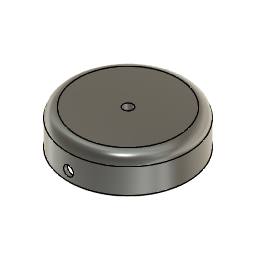
cap tesla coil (Autodesk Fusion 360 design; units mm, degrees)
Autodesk Fusion 360 part; units mm, degrees
sketch "Sketch1" plane through (0, 0, 0) normal (0, 0, 1) x (1, 0, 0)
  circle A0 centre (0, 0) radius 23
  circle A1 centre (0, 0) radius 24.5
  dimension "d1" = 46
  dimension "d2" = 49
  constraint coincident A0.centre A1.centre
  measures "d1" diameter of A0
  measures "d2" diameter of A1
extrude "Extrude1" add sketch "Sketch1" along normal blind 12
sketch "Sketch2" plane through (0, 0, 12) normal (0, 0, 1) x (-1, 0, 0)
  circle A0 centre (0, 0) radius 23
  circle A1 centre (0, 0) radius 24.5
  circle A2 centre (0, 0) radius 2
  circle A3 centre (0, 0) radius 24.5
  dimension "d5" = 4
  constraint coincident A0.centre A1.centre
  measures "d5" diameter of A2
extrude "Extrude2" add sketch "Sketch2" along normal blind 3 contours A0 | A1 A3
fillet "Fillet1" radius 4 1 edges at (22.842, 8.8596, 15)
sketch "Sketch3" plane through (0, 0, 0) normal (0, 1, 0) x (1, 0, 0)
  line L0 (0, 0) -> (0, -4.5)
  circle A0 centre (0, -4.5) radius 2
  dimension "d10" = 4.5
  dimension "d11" = 4
  constraint coincident L0.start origin
  constraint vertical L0
  constraint coincident L0.end A0.centre
  measures "d10" distance of L0.start L0.end
  measures "d11" diameter of A0
extrude "Extrude3" cut sketch "Sketch3" along normal mid plane 700
fillet "Fillet2" radius 0.75 2 edges at (-22.842, -8.8596, 0) (-21.4435, 8.3172, 0)
